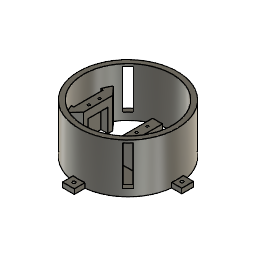
assemblyv3 (Autodesk Fusion 360 archive; units mm, degrees)
design "base"
part number: 2026-03-31-09-29-29-692
Autodesk Fusion 360 part; units mm, degrees
note: some values were not read from the file. Chosen so that the rebuilt part matches the saved one: a direction; which face or edge a step refers to. Set by a fixed rule: which sketch regions a step uses.
sketch "Sketch1" plane through (0, 0, 0) normal (0, 0, 1) x (1, 0, 0)
  circle A0 centre (0, 0) radius 50
  circle A1 centre (0, 0) radius 45
  dimension "d2" = 100
  dimension "d3" = 90
  constraint coincident A0.centre A1.centre
  constraint concentric A0 A1
  measures "d2" diameter of A0
  measures "d3" diameter of A1
extrude "Extrude1" add sketch "Sketch1" along normal blind 50
sketch "Sketch2" plane through (0, 0, 0) normal (0, 0, 1) x (1, 0, 0)
sketch "Sketch3" plane through (0, 0, 0) normal (0, 0, 1) x (1, 0, 0)
  line L0 (45, 10) -> (45, -10)
  line L1 (-39.9643, -25.0714) -> (-30.45, -14.5)
  line L2 (-30.45, -14.5) -> (-30.45, 14.9449)
  line L3 (-30.45, 14.9449) -> (-39.8514, 25.2971)
  line L4 (-39.8514, 25.2971) -> (-45, 15)
  line L5 (-45, 15) -> (-40, 15)
  line L6 (-40, 15) -> (-40, -15)
  line L7 (-40, -15) -> (-45, -15)
  line L8 (-45, -15) -> (-39.9643, -25.0714)
  constraint vertical L0
  constraint vertical L2
  constraint perpendicular L2 L5
  constraint perpendicular L5 L6
  constraint perpendicular L6 L7
extrude "Extrude2" add sketch "Sketch3" along normal blind 31.2
sketch "Sketch4" plane through (0, 0, 0) normal (0, 0, 1) x (1, 0, 0)
  line L0 (-30, -10) -> (-30, 10)
  line L1 (-30, 10) -> (-37.498, 10)
  line L2 (-37.498, 10) -> (-37.498, -10)
  line L3 (-37.498, -10) -> (-30, -10)
  constraint vertical L0
  constraint perpendicular L0 L1
  constraint perpendicular L1 L2
  constraint perpendicular L0 L3
extrude "Extrude3" cut sketch "Sketch4" along normal blind 23.2
sketch "pos" plane through (0, 0, 0) normal (0, 0, 1) x (1, 0, 0)
  circle A0 centre (-34.4411, -5.8081) radius 1.25
  circle A1 centre (-34.4411, -5.8081) radius 1.25
  circle A2 centre (-34.4411, 6.026) radius 1.25
  point P0 (-34.4411, -5.8081)
  point P1 (-34.4411, -5.8081)
  dimension "d12" = 2.5
  dimension "d14" = 2.5
  measures "d12" diameter of A0
  measures "d14" diameter of A2
extrude "Extrude4" cut sketch "pos" along normal blind 31.2
sketch "Sketch6" plane through (0, 0, 0) normal (0, 0, 1) x (1, 0, 0)
  line L0 (30, 35) -> (10, 15)
  line L1 (20, 15) -> (35, 30)
  line L2 (35, 30) -> (30, 35)
  line L3 (35, -30) -> (20, -15)
  line L4 (10, -15) -> (30, -35)
  line L5 (30, -35) -> (35, -30)
  line L6 (20, -15) -> (20, 15)
  line L7 (10, 15) -> (10, -15)
  constraint parallel L0 L1
  constraint perpendicular L0 L2
  constraint perpendicular L0 L3
  constraint perpendicular L0 L4
  constraint perpendicular L3 L5
  constraint vertical L6
  constraint parallel L6 L7
extrude "Extrude5" add sketch "Sketch6" along normal blind 5
sketch "Sketch7" plane through (0, 0, 0) normal (0, 0, 1) x (1, 0, 0)
  line L0 (20, -15) -> (10, -15)
  line L1 (10, -15) -> (10, 15)
  line L2 (10, 15) -> (20, 15)
  line L3 (20, 15) -> (20, -15)
  constraint horizontal L0
  constraint perpendicular L0 L1
  constraint perpendicular L1 L2
  constraint perpendicular L0 L3
extrude "Extrude6" add sketch "Sketch7" along normal blind 31.3
sketch "Sketch8" plane through (0, 0, 0) normal (0, 0, 1) x (1, 0, 0)
  line L0 (10, -10) -> (20, -10)
  line L1 (20, -10) -> (20, 10)
  line L2 (20, 10) -> (10, 10)
  line L3 (10, 10) -> (10, -10)
  constraint horizontal L0
  constraint perpendicular L0 L1
  constraint perpendicular L1 L2
  constraint perpendicular L0 L3
extrude "Extrude7" cut sketch "Sketch8" along normal blind 23.2
sketch "Sketch9" plane through (0, 0, 31.3) normal (0, 0, 1) x (1, 0, 0)
  circle A0 centre (14.3675, 6.0119) radius 1.25
  circle A1 centre (14.3675, -5.7062) radius 1.25
  line L0 (20, 15) -> (10, 15)
  line L1 (10, 15) -> (10, -15)
  line L2 (10, -15) -> (20, -15)
  line L3 (20, -15) -> (20, 15)
  dimension "d23" = 2.5
  dimension "d24" = 2.5
  measures "d23" diameter of A0
  measures "d24" diameter of A1
extrude "Extrude8" cut sketch "Sketch9" along normal blind 32 contours A0 | A1
sketch "Sketch10" plane through (0, 0, 0) normal (0, 0, 1) x (1, 0, 0)
  line L0 (-6, 61) -> (6, 61)
  line L1 (6, 61) -> (6, 49)
  line L2 (6, 49) -> (-6, 49)
  line L3 (-6, 49) -> (-6, 61)
  line L4 (48, 6.6) -> (60, 6.6)
  line L5 (48, -5.4) -> (48, 6.6)
  line L6 (60, 6.6) -> (60, -5.4)
  line L7 (60, -5.4) -> (48, -5.4)
  line L8 (-6, -48.5) -> (6, -48.5)
  line L9 (6, -48.5) -> (6, -60.5)
  line L10 (6, -60.5) -> (-6, -60.5)
  line L11 (-6, -60.5) -> (-6, -48.5)
  line L12 (-48.4367, 6.0382) -> (-48.4367, -5.9618)
  line L13 (-48.4367, -5.9618) -> (-60.4367, -5.9618)
  line L14 (-60.4367, 6.0382) -> (-48.4367, 6.0382)
  line L15 (-60.4367, -5.9618) -> (-60.4367, 6.0382)
  circle A0 centre (0, 55) radius 1.5
  circle A1 centre (0, 55) radius 1.5
  circle A2 centre (54.4367, 0.5633) radius 1.5
  circle A3 centre (0, -54.9236) radius 1.5
  circle A4 centre (-54.6117, -0.3119) radius 1.5
  point P0 (0, 55)
  point P1 (0, 55)
  dimension "d27" = 12
  dimension "d28" = 12
  dimension "d29" = 12
  dimension "d30" = 12
  dimension "d31" = 12
  dimension "d32" = 12
  dimension "d33" = 12
  dimension "d34" = 12
  dimension "d35" = 3
  dimension "d36" = 3
  dimension "d37" = 3
  dimension "d38" = 3
  dimension "d39" = 3
  constraint horizontal L0
  constraint vertical L1
  constraint horizontal L2
  constraint vertical L3
  constraint horizontal L4
  constraint vertical L6
  constraint horizontal L7
  constraint vertical L5
  constraint horizontal L8
  constraint vertical L9
  constraint horizontal L10
  constraint vertical L11
  constraint horizontal L14
  constraint vertical L12
  constraint horizontal L13
  constraint vertical L15
  measures "d27" distance of L0.start L0.end
  measures "d28" distance of L0.start L2.end
  measures "d29" distance of L4.end L4.start
  measures "d30" distance of L5.start L4.start
  measures "d31" distance of L8.end L8.start
  measures "d32" distance of L10.end L8.start
  measures "d33" distance of L12.start L14.start
  measures "d34" distance of L13.end L14.start
  measures "d35" diameter of A0
  measures "d36" diameter of A1
  measures "d37" diameter of A2
  measures "d38" diameter of A3
  measures "d39" diameter of A4
extrude "Extrude9" add sketch "Sketch10" along normal blind 5
sketch "Sketch11" plane through (0, 0, 0) normal (0, 0, 1) x (1, 0, 0)
extrude "Extrude10" add sketch "pos" along normal blind 31.2
extrude "Extrude11" cut sketch "pos" along normal blind 23.2
sketch "Sketch12" plane through (0, 0, 0) normal (0, 0, 1) x (1, 0, 0)
  circle A0 centre (-34.2402, -5.5137) radius 1.2
  circle A1 centre (-34.1643, 5.4157) radius 1.2
  circle A2 centre (14.3038, -5.4861) radius 1.2
  circle A3 centre (14.3038, 5.3812) radius 1.2
  dimension "d46" = 2.4
  dimension "d47" = 2.4
  dimension "d48" = 2.4
  dimension "d49" = 2.4
  measures "d46" diameter of A0
  measures "d47" diameter of A1
  measures "d48" diameter of A2
  measures "d49" diameter of A3
extrude "Extrude12" cut sketch "Sketch12" along normal blind 32
ref_plane "WorkPlane1" through (35.3553, 35.3553, 38.0932) normal (0.707107, 0.707107, 0) x (0.707107, -0.707107, 0)
sketch "Sketch13" plane through (35.3553, 35.3553, 0) normal (0.707107, 0.707107, 0) x (-0.707107, 0.707107, 0)
  line L0 (-3.75, 47.3778) -> (3.75, 47.3778)
  line L1 (3.75, 47.3778) -> (3.75, 7.3778)
  line L2 (3.75, 7.3778) -> (-3.75, 7.3778)
  line L3 (-3.75, 7.3778) -> (-3.75, 47.3778)
  dimension "d53" = 7.5
  dimension "d54" = 40
  constraint horizontal L0
  constraint vertical L1
  constraint horizontal L2
  constraint vertical L3
  measures "d53" distance of L0.start L0.end
  measures "d54" distance of L0.start L2.end
extrude "Extrude13" cut sketch "Sketch13" against normal blind 5.2
pattern_circular "C-Pattern1" count 4 over 360 about axis through (0, 0, 1.75) along (0, 0, 1) of "Extrude13"
equation "baseRadius = 50 mm"
equation "d2 = 2 * baseRadius"
equation "d3 = 2 * ( baseRadius - 5 mm )"
equation "baseHeight = 50 mm"
equation "d5 = baseHeight"
equation "d8 = 50 mm - 18.8 mm"
equation "d21 = 31.2 mm - 8 mm"
equation "d44 = 31.2 mm - 8 mm"

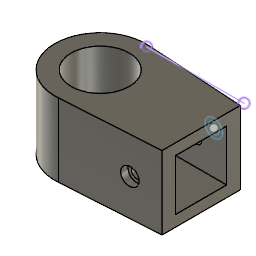
design "arm11"
part number: 2026-03-31-18-45-55-924
Autodesk Fusion 360 part; units mm, degrees
sketch "Sketch1" plane through (0, 0, 0) normal (0, 0, 1) x (1, 0, 0)
  circle A0 centre (0, 0) radius 11.5
  circle A1 centre (0, 0) radius 18
  line L0 (0.8567, 17.9796) -> (40, 15.5)
  line L1 (40, 15.5) -> (40, -15.5)
  line L2 (40, -15.5) -> (1.4283, -17.9432)
  line L3 (1.75, 0) -> (22.5, 0)
  circle A2 centre (4.4, 0) radius 0.725
  circle A3 centre (4.4, 0) radius 0.725
  circle A4 centre (-4.4, 0) radius 0.725
  circle A5 centre (0, 5.3) radius 0.725
  circle A6 centre (0, -5.3) radius 0.725
  dimension "d1" = 23
  dimension "d2" = 31
  dimension "d3" = 40
  dimension "d4" = 36
  dimension "d15" = 1.45
  dimension "d16" = 4.4
  dimension "d17" = 1.45
  dimension "d18" = 1.45
  dimension "d19" = 4.4
  dimension "d20" = 1.45
  dimension "d21" = 1.45
  constraint coincident A0.centre A1.centre
  constraint coincident A1 L0.start
  constraint vertical L1
  constraint coincident A1 L2.end
  constraint symmetric L0.end L1.end L3
  constraint coincident L3 A2.centre
  measures "d1" diameter of A0
  measures "d2" distance of L0.end L1.end
  measures "d3" distance of A0.centre L1
  measures "d4" diameter of A1
  measures "d15" diameter of A2
  measures "d16" distance of A0.centre A2.centre
  measures "d17" diameter of A3
  measures "d18" diameter of A4
  measures "d19" distance of A0.centre A4.centre
  measures "d20" diameter of A5
  measures "d21" diameter of A6
extrude "Extrude1" add sketch "Sketch1" along normal blind 29 contours A1 | A1 L0 L1 L2
extrude "Extrude2" add sketch "Sketch1" along normal blind 5 contours A0
sketch "Sketch2" plane through (40, 0, 0) normal (1, 0, 0) x (0, 1, 0)
  line L0 (-15.5, 0) -> (15.5, 0)
  line L1 (15.5, 0) -> (15.5, 29)
  line L2 (15.5, 29) -> (-15.5, 29)
  line L3 (-15.5, 29) -> (-15.5, 0)
  line L4 (-10.1, 24.6) -> (10.1, 24.6)
  line L5 (10.1, 24.6) -> (10.1, 4.4)
  line L6 (10.1, 4.4) -> (-10.1, 4.4)
  line L7 (-10.1, 4.4) -> (-10.1, 24.6)
  line L8 (15.5, 0) -> (-15.5, 0)
  dimension "d9" = 20.2
  dimension "d10" = 20.2
  dimension "d11" = 4.4
  dimension "d12" = 5.4
  constraint horizontal L4
  constraint vertical L5
  constraint horizontal L6
  constraint vertical L7
  measures "d9" distance of L4.start L4.end
  measures "d10" distance of L4.start L6.end
  measures "d11" distance of L6 L8
  measures "d12" distance of L3 L7
extrude "Extrude3" cut sketch "Sketch2" against normal blind 20 contours L4 L5 L6 L7
sketch "Sketch3" plane through (0, 0, 0) normal (0, 1, 0) x (1, 0, 0)
  circle A0 centre (28, -14.5) radius 3.45
  line L0 (0.8567, 0) -> (40, 0)
  line L1 (40, 0) -> (40, -29)
  circle A1 centre (28, -14.5) radius 2.1
  dimension "d22" = 6.9
  dimension "d23" = 14.5
  dimension "d24" = 12
  dimension "d25" = 4.2
  constraint concentric A0 A1
  measures "d22" diameter of A0
  measures "d23" distance of A0.centre L0
  measures "d24" distance of A0.centre L1
  measures "d25" diameter of A1
ref_plane "WorkPlane2" through (28, 17, 14.5) normal (0, 1, 0) x (1, 0, 0)
sketch "Sketch4" plane through (0, 17, 0) normal (0, 1, 0) x (1, 0, 0)
  circle A0 centre (28, -14.5) radius 2.1
  circle A1 centre (28, -14.5) radius 3.45
  line L0 (1.4283, -29) -> (40, -29)
  dimension "d28" = 4.2
  dimension "d29" = 6.9
  dimension "d39" = 14.5
  constraint concentric A0 A1
  measures "d28" diameter of A0
  measures "d29" diameter of A1
  measures "d39" distance of A0.centre L0
extrude "Extrude4" cut sketch "Sketch4" against normal blind 35 contours A0
extrude "Extrude5" cut sketch "Sketch4" against normal blind 3.4
ref_plane "WorkPlane3" through (0, -17, 0) normal (0, 1, 0) x (1, 0, 0)
sketch "Sketch5" plane through (0, -17, 0) normal (0, 1, 0) x (1, 0, 0)
  circle A0 centre (28, -14.5) radius 2.1
  circle A1 centre (28, -14.5) radius 3.45
  line L0 (1.4283, -29) -> (40, -29)
  dimension "d35" = 4.2
  dimension "d36" = 6.9
  dimension "d40" = 14.5
  constraint concentric A0 A1
  measures "d35" diameter of A0
  measures "d36" diameter of A1
  measures "d40" distance of A0.centre L0
extrude "Extrude6" cut sketch "Sketch5" along normal blind 3.4
equation "d11 = ( 29 / 2 ) * 1 mm - ( 20.2 / 2 ) * 1 mm"
equation "d12 = ( 31 / 2 ) * 1 mm - ( 20.2 / 2 ) * 1 mm"
equation "d23 = ( 29 / 2 ) * 1 mm"

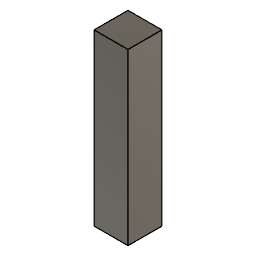
design "alRod"
part number: 2026-04-02-00-39-57-906
Autodesk Fusion 360 part; units mm, degrees
sketch "Sketch1" plane through (0, 0, 0) normal (0, 0, 1) x (1, 0, 0)
  line L0 (-10, 10) -> (10, 10)
  line L1 (10, 10) -> (10, -10)
  line L2 (10, -10) -> (-10, -10)
  line L3 (-10, -10) -> (-10, 10)
  constraint horizontal L0
  constraint vertical L1
  constraint horizontal L2
  constraint vertical L3
extrude "Extrude1" add sketch "Sketch1" along normal blind 100

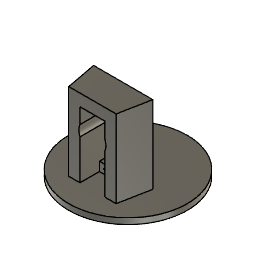
design "baseCover"
part number: 2026-03-31-10-25-44-366
Autodesk Fusion 360 part; units mm, degrees
sketch "Sketch1" plane through (0, 0, 0) normal (0, 0, 1) x (1, 0, 0)
  circle A0 centre (0, 0) radius 50
  circle A1 centre (4.4, 0) radius 0.725
  circle A2 centre (-4.4, 0) radius 0.725
  circle A3 centre (0, 5.3) radius 0.725
  dimension "d2" = 100
  dimension "d3" = 1.45
  dimension "d4" = 4.4
  dimension "d5" = 1.45
  dimension "d6" = 4.4
  dimension "d29" = 1.45
  dimension "d30" = 5.3
  constraint coincident A0.centre origin
  measures "d2" diameter of A0
  measures "d3" diameter of A1
  measures "d4" distance of A0.centre A1.centre
  measures "d5" diameter of A2
  measures "d6" distance of A0.centre A2.centre
  measures "d29" diameter of A3
  measures "d30" distance of A0.centre A3.centre
extrude "Extrude1" add sketch "Sketch1" along normal blind 5
sketch "Sketch2" plane through (0, 0, 5) normal (0, 0, 1) x (-1, 0, 0)
  circle A0 centre (-4.4, 0) radius 0.725
  circle A1 centre (4.4, 0) radius 0.725
  circle A2 centre (0, 0) radius 50
  line L0 (25, 4) -> (-25, 4)
  line L1 (-25, 4) -> (25, 4)
  line L2 (25, 4) -> (20, 30)
  line L3 (20, 30) -> (-20, 30)
  line L4 (-20, 30) -> (-25, 4)
  circle A3 centre (0, -5.3) radius 0.725
  constraint horizontal L0
extrude "Extrude2" add sketch "Sketch2" along normal blind 65.5 contours L0 L1 L2 L3 L4
sketch "Sketch4" plane through (0, -24, 0) normal (0, -1, 0) x (1, 0, 0)
  line L0 (21.1538, 5) -> (25, 5)
  line L1 (25, 5) -> (25, 70.5)
  line L2 (25, 70.5) -> (21.1538, 70.5)
  circle A0 centre (-0.1, 43) radius 11.526
  line L3 (21.1538, 70.5) -> (21.1538, 5)
sketch "Sketch5" plane through (0, -30, 0) normal (0, -1, 0) x (1, 0, 0)
  line L0 (-20, 5) -> (20, 5)
  line L1 (20, 5) -> (20, 70.5)
  line L2 (20, 70.5) -> (-20, 70.5)
  line L3 (-20, 70.5) -> (-20, 5)
  circle A0 centre (0, 43) radius 11.4182
extrude "Extrude4" cut sketch "Sketch5" against normal blind 27 contours A0
sketch "Sketch6" plane through (0, -30, 0) normal (0, -1, 0) x (1, 0, 0)
  circle A0 centre (0, 43) radius 11.4182
  line L0 (-20, 5) -> (20, 5)
  line L1 (20, 5) -> (20, 70.5)
  line L2 (20, 70.5) -> (-20, 70.5)
  line L3 (-20, 70.5) -> (-20, 5)
  line L4 (-10.5, 60.5) -> (10.5, 60.5)
  line L5 (10.5, 60.5) -> (10.5, 5)
  line L6 (10.5, 5) -> (-10.5, 5)
  line L7 (-10.5, 5) -> (-10.5, 60.5)
  line L8 (-1.072, 60.5) -> (1, 60.5)
  line L9 (1, 60.5) -> (1, 53)
  line L10 (1, 53) -> (-1.072, 53)
  line L11 (-1.072, 53) -> (-1.072, 60.5)
  line L12 (-1, 5) -> (1, 5)
  line L13 (1, 5) -> (1, 14)
  line L14 (1, 14) -> (-1, 14)
  line L15 (-1, 14) -> (-1, 5)
  circle A1 centre (-5.5975, 57.2496) radius 1.2
  circle A2 centre (5.3042, 57.2496) radius 1.2
  circle A3 centre (-5.5975, 8.6679) radius 1.2
  circle A4 centre (5.3751, 8.6305) radius 1.2
  dimension "d21" = 2.4
  dimension "d22" = 2.4
  dimension "d23" = 2.4
  dimension "d24" = 2.4
  constraint horizontal L4
  constraint vertical L5
  constraint horizontal L6
  constraint vertical L7
  constraint coincident L0 L5.end
  constraint horizontal L8
  constraint vertical L9
  constraint horizontal L10
  constraint vertical L11
  constraint coincident L4 L8.start
  constraint horizontal L12
  constraint vertical L13
  constraint horizontal L14
  constraint vertical L15
  constraint coincident L0 L12.start
  measures "d21" diameter of A1
  measures "d22" diameter of A2
  measures "d23" diameter of A3
  measures "d24" diameter of A4
extrude "Extrude5" cut sketch "Sketch6" against normal blind 16.4 contours A0 L4 L5 L9 | A0 L0 L5 L6 L7 L13 L14 L15 | A0 L4 L7 L11 | A1 | A2 | A3 | A4
extrude "Extrude6" cut sketch "Sketch6" against normal blind 19.5 contours A0 L4 L8 L9 L11 | L0 L6 L12 L13 L14 L15
extrude "Extrude7" cut sketch "Sketch6" against normal blind 21.4 contours A1 | A2 | A3 | A4
sketch "Sketch7" plane through (0, -30, 0) normal (0, -1, 0) x (1, 0, 0)
  line L0 (-10.5, 60.5) -> (10.5, 60.5)
  line L1 (10.5, 60.5) -> (10.5, 47.4862)
  arc A0 (10.5, 38.5138) -> (10.5, 47.4862) centre (0, 43) ccw
  line L2 (10.5, 38.5138) -> (10.5, 5)
  line L3 (10.5, 5) -> (20, 5)
  line L4 (20, 5) -> (20, 70.5)
  line L5 (20, 70.5) -> (-20, 70.5)
  line L6 (-20, 70.5) -> (-20, 5)
  line L7 (-20, 5) -> (-10.5, 5)
  line L8 (-10.5, 5) -> (-10.5, 38.5138)
  arc A1 (-10.5, 47.4862) -> (-10.5, 38.5138) centre (0, 43) ccw
  line L9 (-10.5, 47.4862) -> (-10.5, 60.5)
  line L10 (10.5, 53.9931) -> (-10.5, 53.9931)
  line L11 (-10.5, 53.9931) -> (-10.5, 12.5264)
  line L12 (-10.5, 12.5264) -> (10.5, 12.5264)
  line L13 (10.5, 12.5264) -> (10.5, 53.9931)
  constraint horizontal L10
  constraint vertical L11
  constraint horizontal L12
  constraint vertical L13
  constraint coincident L8 L11.end
  constraint midpoint L1 L10.start
extrude "Extrude8" cut sketch "Sketch7" against normal blind 25 contours L1 L2 L8 L9 L10 L11 L12 L13
sketch "Sketch8" plane through (0, -30, 0) normal (0, -1, 0) x (1, 0, 0)
  line L0 (-10.5, 60.5) -> (10.5, 60.5)
  line L1 (10.5, 60.5) -> (10.5, 47.4862)
  arc A0 (10.5, 38.5138) -> (10.5, 47.4862) centre (0, 43) ccw
  line L2 (10.5, 38.5138) -> (10.5, 5)
  line L3 (10.5, 5) -> (20, 5)
  line L4 (20, 5) -> (20, 70.5)
  line L5 (20, 70.5) -> (-20, 70.5)
  line L6 (-20, 70.5) -> (-20, 5)
  line L7 (-20, 5) -> (-10.5, 5)
  line L8 (-10.5, 5) -> (-10.5, 38.5138)
  arc A1 (-10.5, 47.4862) -> (-10.5, 38.5138) centre (0, 43) ccw
  line L9 (-10.5, 47.4862) -> (-10.5, 60.5)
equation "baseRadius = 50 mm"
equation "d2 = 2 * baseRadius"
equation "d17 = -30 mm + 13.6 mm"
equation "d25 = -16.4 mm - 5 mm"
equation "d27 = -17.4 mm - 7.6 mm"

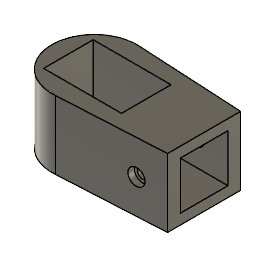
design "arm21"
part number: 2026-03-31-18-45-55-924
Autodesk Fusion 360 part; units mm, degrees
sketch "Sketch1" plane through (0, 0, 0) normal (0, 0, 1) x (1, 0, 0)
  circle A0 centre (0, 0) radius 18
  line L0 (0.8557, 17.9796) -> (46.5, 15.5)
  line L1 (46.5, 15.5) -> (46.5, -15.5)
  line L2 (46.5, -15.5) -> (1.4272, -17.9433)
  line L3 (1.75, 0) -> (22.5, 0)
  dimension "d2" = 31
  dimension "d3" = 46.5
  dimension "d4" = 36
  constraint coincident A0.centre origin
  constraint coincident A0 L0.start
  constraint vertical L1
  constraint coincident A0 L2.end
  constraint symmetric L0.end L1.end L3
  measures "d2" distance of L0.end L1.end
  measures "d3" distance of A0.centre L1
  measures "d4" diameter of A0
extrude "Extrude1" add sketch "Sketch1" along normal blind 29
sketch "Sketch2" plane through (46.5, 0, 0) normal (1, 0, 0) x (0, 1, 0)
  line L0 (-15.5, 0) -> (15.5, 0)
  line L1 (15.5, 0) -> (15.5, 29)
  line L2 (15.5, 29) -> (-15.5, 29)
  line L3 (-15.5, 29) -> (-15.5, 0)
  line L4 (-10.1, 24.6) -> (10.1, 24.6)
  line L5 (10.1, 24.6) -> (10.1, 4.4)
  line L6 (10.1, 4.4) -> (-10.1, 4.4)
  line L7 (-10.1, 4.4) -> (-10.1, 24.6)
  line L8 (15.5, 0) -> (-15.5, 0)
  dimension "d9" = 20.2
  dimension "d10" = 20.2
  dimension "d11" = 4.4
  dimension "d12" = 5.4
  constraint horizontal L4
  constraint vertical L5
  constraint horizontal L6
  constraint vertical L7
  measures "d9" distance of L4.start L4.end
  measures "d10" distance of L4.start L6.end
  measures "d11" distance of L6 L8
  measures "d12" distance of L3 L7
extrude "Extrude3" cut sketch "Sketch2" against normal blind 20 contours L4 L5 L6 L7
sketch "S5" plane through (0, 0, 0) normal (0, 0, 1) x (1, 0, 0)
  line L0 (20, 70.5) -> (-20, 70.5)
  line L1 (-20, 70.5) -> (-20, 5)
  line L2 (20, 5) -> (20, 70.5)
  line L3 (-20, 5) -> (20, 5)
  circle A0 centre (0, 43) radius 11.4182
sketch "S6" plane through (0, 0, 0) normal (0, 0, 1) x (1, 0, 0)
  circle A0 centre (0, 43) radius 11.4182
  line L0 (20, 5) -> (20, 70.5)
  line L1 (-20, 70.5) -> (-20, 5)
  line L2 (-20, 5) -> (20, 5)
  line L3 (20, 70.5) -> (-20, 70.5)
  line L4 (10.5, 60.5) -> (10.5, 5)
  line L5 (-10.5, 60.5) -> (10.5, 60.5)
  line L6 (-10.5, 5) -> (-10.5, 60.5)
  line L7 (10.5, 5) -> (-10.5, 5)
  line L8 (-1.072, 60.5) -> (1, 60.5)
  line L9 (1, 53) -> (-1.072, 53)
  line L10 (1, 60.5) -> (1, 53)
  line L11 (-1.072, 53) -> (-1.072, 60.5)
  line L12 (1, 5) -> (1, 14)
  line L13 (1, 14) -> (-1, 14)
  line L14 (-1, 14) -> (-1, 5)
  line L15 (-1, 5) -> (1, 5)
  circle A1 centre (-5.5975, 57.2496) radius 1.2
  circle A2 centre (5.3042, 57.2496) radius 1.2
  circle A3 centre (-5.5975, 8.6679) radius 1.2
  circle A4 centre (5.3751, 8.6305) radius 1.2
sketch "S7" plane through (0, 0, 0) normal (0, 0, 1) x (1, 0, 0)
  line L0 (-10.5, 47.4862) -> (-10.5, 60.5)
  line L1 (-20, 70.5) -> (-20, 5)
  arc A0 (10.5, 47.4862) -> (10.5, 38.5138) centre (0, 43) cw
  arc A1 (-10.5, 38.5138) -> (-10.5, 47.4862) centre (0, 43) cw
  line L2 (-20, 5) -> (-10.5, 5)
  line L3 (-10.5, 5) -> (-10.5, 38.5138)
  line L4 (10.5, 60.5) -> (10.5, 47.4862)
  line L5 (10.5, 5) -> (20, 5)
  line L6 (-10.5, 60.5) -> (10.5, 60.5)
  line L7 (10.5, 38.5138) -> (10.5, 5)
  line L8 (20, 5) -> (20, 70.5)
  line L9 (20, 70.5) -> (-20, 70.5)
  line L10 (-10.5, 53.9931) -> (-10.5, 12.5264)
  line L11 (-10.5, 12.5264) -> (10.5, 12.5264)
  line L12 (10.5, 53.9931) -> (-10.5, 53.9931)
  line L13 (10.5, 12.5264) -> (10.5, 53.9931)
sketch "Sketch6" plane through (0, 0, 29) normal (0, 0, 1) x (1, 0, 0)
  circle A0 centre (0, 0) radius 6.6465
  line L0 (21.99, -10.5) -> (21.99, 10.5)
  line L1 (-8.3709, 10.5) -> (21.99, 10.5)
  line L2 (21.99, 10.5) -> (21.99, -10.5)
  circle A1 centre (-8.1, 0.1007) radius 1.2
  circle A2 centre (19.45, 0) radius 1.2
  line L3 (-6.7, 6.9) -> (11.3, 6.9)
  line L4 (-6.7, -7.1) -> (-6.7, 6.9)
  line L5 (11.3, 6.9) -> (11.3, -7.1)
  line L6 (11.3, -7.1) -> (-6.7, -7.1)
  line L7 (21.99, -10.5) -> (-7.5099, -10.5)
  line L8 (-18.0099, 0) -> (-18.0099, 0.0354)
  line L9 (21.99, 10.5354) -> (21.99, -10.5)
  line L10 (46.5, 15.5) -> (0.8557, 17.9796)
  arc A3 (0.8557, 17.9796) -> (1.4272, -17.9433) centre (0, 0) ccw
  line L11 (1.4272, -17.9433) -> (46.5, -15.5)
  line L12 (46.5, -15.5) -> (46.5, 15.5)
  line L13 (21.99, 10.5) -> (-11.01, 10.5)
  line L14 (-11.01, 10.5) -> (-11.01, -10.5)
  line L15 (-11.01, -10.5) -> (21.99, -10.5)
  line L16 (21.99, -10.5) -> (21.99, 10.5)
  dimension "d15" = 33
  dimension "d16" = 21
  dimension "d17" = 18
  constraint horizontal L13
  constraint vertical L14
  constraint horizontal L15
  constraint vertical L16
  constraint coincident L1 L0.end
  measures "d15" distance of L0.end L13.end
  measures "d16" distance of L0.end L0.start
  measures "d17" distance of L4 L5
extrude "Extrude4" cut sketch "Sketch6" against normal blind 29.5 contours A0 | L3 L4 L5 L6
extrude "Extrude5" cut sketch "Sketch6" against normal blind 21.5 contours A0 | L0 L1 L2 L7 L9 L13 L14 L15 L16 | L3 L4 L5 L6
extrude "Extrude6" cut sketch "Sketch6" against normal blind 26.5 contours A1 | A2
sketch "tboltholes" plane through (0, 0, 0) normal (0, 1, 0) x (1, 0, 0)
  circle A0 centre (34, -14.5) radius 3.45
  line L0 (0.8567, 0) -> (40, 0)
  line L1 (40, 0) -> (40, -29)
  circle A1 centre (34, -14.5) radius 2.1
  line L2 (46.5, 0) -> (46.5, -29)
  line L3 (1.4272, -29) -> (46.5, -29)
  dimension "d24" = 12.5
  dimension "d25" = 12.5
  dimension "d26" = 14.5
  constraint coincident A0.centre A1.centre
  measures "d24" distance of A0.centre L2
  measures "d25" distance of A0.centre L2
  measures "d26" distance of A0.centre L3
ref_plane "WorkPlane1" through (0, 17, 0) normal (0, 1, 0) x (1, 0, 0)
ref_plane "WorkPlane2" through (0, -17, 0) normal (0, 1, 0) x (1, 0, 0)
sketch "Sketch9" plane through (0, 17, 0) normal (0, 1, 0) x (1, 0, 0)
  circle A0 centre (34, -14.5) radius 2.1
  circle A1 centre (34, -14.5) radius 3.45
  dimension "d29" = 4.2
  dimension "d30" = 6.9
  constraint concentric A0 A1
  measures "d29" diameter of A0
  measures "d30" diameter of A1
sketch "Sketch10" plane through (0, -17, 0) normal (0, 1, 0) x (1, 0, 0)
  circle A0 centre (34, -14.5) radius 2.1
  circle A1 centre (34, -14.5) radius 3.45
  dimension "d31" = 4.2
  dimension "d32" = 6.9
  constraint concentric A0 A1
  measures "d31" diameter of A0
  measures "d32" diameter of A1
extrude "Extrude7" cut sketch "Sketch10" along normal blind 35 contours A0
extrude "Extrude8" cut sketch "Sketch10" along normal blind 3.4
extrude "Extrude9" cut sketch "Sketch9" against normal blind 3.4
sketch "Sketch11" plane through (0, 0, 0) normal (0, 0, -1) x (1, 0, 0)
  line L0 (11.3, -6.9) -> (-6.7, -6.9)
  line L1 (-6.7, -6.9) -> (-6.7, 7.1)
  line L2 (-6.7, 7.1) -> (11.3, 7.1)
  line L3 (11.3, 7.1) -> (11.3, -6.9)
  line L4 (0.8557, -17.9796) -> (46.5, -15.5)
  line L5 (46.5, -15.5) -> (46.5, 15.5)
  line L6 (46.5, 15.5) -> (1.4272, 17.9433)
  arc A0 (1.4272, 17.9433) -> (0.8557, -17.9796) centre (0, 0) ccw
  line L7 (-0.0048, 7.1) -> (-0.0048, 0.1)
  dimension "d39" = 7
  constraint coincident L2 L7.start
  constraint perpendicular L2 L7
  measures "d39" distance of L7.start L7.end
equation "d3 = 50 mm - 3.5 mm"
equation "d11 = ( 29 / 2 ) * 1 mm - ( 20.2 / 2 ) * 1 mm"
equation "d20 = -( 29 mm - 7.5 mm )"
equation "d22 = -( 29 mm - 7.5 mm + 5 mm )"
